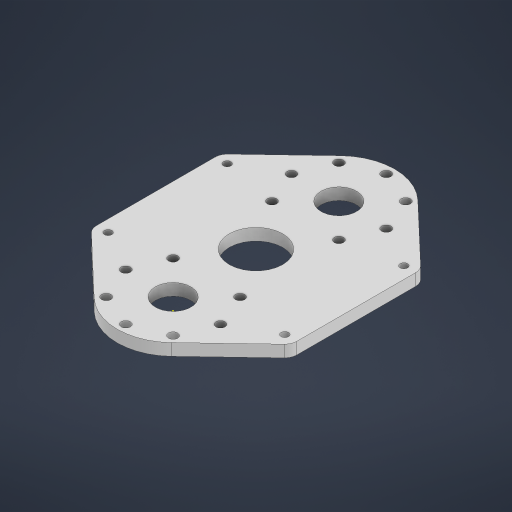
# Autodesk Inventor part: Bottom Plate
Saved by Autodesk Inventor 2024.3 (Build 283343000, 343)
## iProperties
Created: 2024-07-07
Part Number: Bottom Plate
Material: Generic
Document SubType Name: Modeling
Designer: kaito
Density: 1 g/cm^3
Appearance: Default
Author: kaito
Autodesk Inventor part; units mm, degrees
note: some values were not read from the file. Chosen so that the rebuilt part matches the saved one: second side of "Extrusion1".
ref_plane "YZ Plane" through (0, 0, 0) normal (1, 0, 0) x (0, 1, 0)
ref_plane "XZ Plane" through (0, 0, 0) normal (0, 1, 0) x (-1, 0, 0)
ref_plane "XY Plane" through (0, 0, 0) normal (0, 0, 1) x (1, 0, 0)
sketch "Sketch1" plane through (0, 0, 0) normal (0, 1, 0) x (-1, 0, 0)
  point P0 (0, 0)
sketch "Sketch2" plane through (0, 0, 0) normal (0, 1, 0) x (-1, 0, 0)
  circle A0 centre (0, 0) radius 6.35 construction
  circle A1 centre (0, -44.45) radius 38.1 construction
  circle A2 centre (0, 0) radius 25.4 construction
  circle A3 centre (17.9605, -17.9605) radius 2.4892
  circle A4 centre (25.4, 0) radius 2.4892
  circle A5 centre (17.9605, 17.9605) radius 2.4892
  circle A6 centre (0, 25.4) radius 2.4892
  circle A7 centre (-17.9605, 17.9605) radius 2.4892
  circle A8 centre (-25.4, 0) radius 2.4892
  circle A9 centre (-17.9605, -17.9605) radius 2.4892
  circle A10 centre (0, -25.4) radius 2.4892 construction
  circle A11 centre (0, -88.9) radius 25.4 construction
  circle A12 centre (0, -88.9) radius 6.35 construction
  circle A13 centre (-17.9605, -70.9395) radius 2.4892
  circle A14 centre (-25.4, -88.9) radius 2.4892
  circle A15 centre (-17.9605, -106.8605) radius 2.4892
  circle A16 centre (0, -114.3) radius 2.4892
  circle A17 centre (17.9605, -106.8605) radius 2.4892
  circle A18 centre (25.4, -88.9) radius 2.4892
  circle A19 centre (17.9605, -70.9395) radius 2.4892
  circle A20 centre (0, -63.5) radius 2.4892 construction
  circle A21 centre (0, 0) radius 9.525
  circle A22 centre (0, -88.9) radius 9.525
  circle A23 centre (47.3968, -12.5178) radius 6.35 construction
  circle A24 centre (47.3968, -76.3822) radius 6.35 construction
  circle A25 centre (-47.3968, -76.3822) radius 6.35 construction
  circle A26 centre (0, 0) radius 29.972 construction
  circle A27 centre (0, -88.9) radius 29.972 construction
  circle A28 centre (-47.3968, -12.5178) radius 6.35 construction
  circle A29 centre (47.3968, -12.5178) radius 2.0193
  circle A30 centre (47.3968, -76.3822) radius 2.0193
  circle A31 centre (-47.3968, -12.5178) radius 2.0193
  circle A32 centre (-47.3968, -76.3822) radius 2.0193
  line L0 (42.1305, -72.8341) -> (31.5979, -65.7381) construction
  line L1 (41.2573, -78.0036) -> (28.9784, -81.2466) construction
  line L2 (-41.2573, -78.0036) -> (-28.9784, -81.2466) construction
  line L3 (-42.1305, -72.8341) -> (-31.5979, -65.7381) construction
  line L4 (-41.2573, -10.8964) -> (-28.9784, -7.6534) construction
  line L5 (-42.1305, -16.0659) -> (-31.5979, -23.1619) construction
  line L6 (41.2573, -10.8964) -> (28.9784, -7.6534) construction
  line L7 (42.1305, -16.0659) -> (31.5979, -23.1619) construction
  line L8 (-20.6699, 21.7043) -> (-51.7761, -7.9195)
  line L9 (-53.7468, -12.5178) -> (-53.7468, -76.3822)
  line L10 (-51.7761, -80.9805) -> (-20.6699, -110.6043)
  line L11 (20.6699, -110.6043) -> (51.7761, -80.9805)
  line L12 (53.7468, -76.3822) -> (53.7468, -12.5178)
  line L13 (51.7761, -7.9195) -> (20.6699, 21.7043)
  arc A33 (20.6699, 21.7043) -> (-20.6699, 21.7043) centre (0, 0) ccw
  arc A34 (-51.7761, -7.9195) -> (-53.7468, -12.5178) centre (-47.3968, -12.5178) ccw
  arc A35 (-53.7468, -76.3822) -> (-51.7761, -80.9805) centre (-47.3968, -76.3822) ccw
  arc A36 (-20.6699, -110.6043) -> (20.6699, -110.6043) centre (0, -88.9) ccw
  arc A37 (51.7761, -80.9805) -> (53.7468, -76.3822) centre (47.3968, -76.3822) ccw
  arc A38 (53.7468, -12.5178) -> (51.7761, -7.9195) centre (47.3968, -12.5178) ccw
  circle A39 centre (0, -44.45) radius 14.351
  dimension "d2" = 50.8
  dimension "d0" = 12.7
  dimension "d1" = 76.2
  dimension "d3" = 4.9784
  dimension "d6" = 360
  dimension "d8" = 4.9784
  dimension "d11" = 360
  dimension "d13" = 19.05
  dimension "d14" = 19.05
  dimension "d15" = 59.944
  dimension "d16" = 59.944
  dimension "d17" = 12.7
  dimension "d18" = 4.0386
  dimension "d24" = 12.7
  dimension "d25" = 28.702
  constraints: 44 point on circle, 38 centre point, 28 end point, 18 tangent, 16 point on line, 12 coincident, 11 equal radius, 7 equal length, 4 vertical alignment, 40 other
  measures "d0" diameter of A0
  measures "d1" diameter of A1
  measures "d3" diameter of A3
  measures "d8" diameter of A13
  measures "d13" diameter of A21
  measures "d14" diameter of A22
  measures "d15" diameter of A26
  measures "d16" diameter of A27
  measures "d17" diameter of A23
  measures "d18" diameter of A29
  measures "d24" distance of L0.start L0.end
  measures "d25" diameter of A39
extrude "Extrusion1" add sketch "Sketch2" along normal blind 6.35
body "Solid1"
